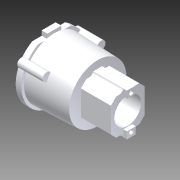
# Autodesk Inventor part: Gear housing BD drill motor
Saved by Autodesk Inventor 2012 (Build 160160000, 160)
## iProperties
Created: 2012-06-30
Part Number: Gear housing BD drill motor
Material: Default
Document SubType Name: Modeling
Designer: Bruce
Density: 1 g/cm^3
Author: Bruce
Autodesk Inventor part; units mm, degrees
ref_plane "YZ Plane" through (0, 0, 0) normal (1, 0, 0) x (0, 1, 0)
ref_plane "XZ Plane" through (0, 0, 0) normal (0, 1, 0) x (-1, 0, 0)
ref_plane "XY Plane" through (0, 0, 0) normal (0, 0, 1) x (1, 0, 0)
sketch "Sketch1" plane through (0, 0, 0) normal (0, 0, 1) x (1, 0, 0)
  line L0 (-46.094, 0) -> (-12.2454, 0)
  line L1 (-12.2454, 0) -> (-12.2454, 20.3708)
  line L2 (-12.2454, 20.3708) -> (-43.1064, 21.5265)
  line L3 (-43.1064, 21.5265) -> (-43.1064, 23.4315)
  line L4 (-43.1064, 23.4315) -> (-47.1704, 23.4315)
  line L5 (-47.1704, 23.4315) -> (-47.1704, 0)
  line L6 (-47.1704, 0) -> (-45.5559, 0)
  point P0 (0, 0)
  dimension "d0" = 4.064
  dimension "d1" = 1.905
  dimension "d2" = 23.4315
  dimension "d3" = 34.925
  dimension "d4" = 20.3708
  dimension "d15" = 0
  constraints: 14 end point, 2 parallel, 2 perpendicular, 1 horizontal, 1 point on line
  measures "d0" distance of L3.end L4.end
  measures "d1" distance of L2.end L3.end
  measures "d2" distance of L4.end L5.end
  measures "d3" distance between parallel lines of L1 L5
  measures "d4" distance of L0.end L1.end
  measures "d15" distance from line of point (0, 0) L0
revolve "Revolution1" add sketch "Sketch1" angle 360 about axis through (-46.094, 0, 0) along (1, 0, 0)
sketch "Sketch2" plane through (-47.1704, 0, 0) normal (-1, 0, 0) x (0, 0, 1)
  circle A0 centre (0, 0) radius 23.4315 projected
  circle A1 centre (0, 0) radius 22.3393 construction
  circle A2 centre (0, -22.3393) radius 3.048
  circle A3 centre (-19.355, 11.1548) radius 3.048
  circle A4 centre (19.355, 11.1548) radius 3.048
  circle A5 centre (-19.355, 11.1548) radius 1.6917
  circle A6 centre (19.355, 11.1548) radius 1.6917
  circle A7 centre (0, -22.3393) radius 1.7363
  line L0 (-11.6676, 20.32) -> (11.6676, 20.32)
  line L1 (11.6676, 20.32) -> (11.6676, 23.6728)
  line L2 (11.6676, 23.6728) -> (-11.6676, 23.6728)
  line L3 (-11.6676, 23.6728) -> (-11.6676, 20.32)
  line L4 (-4.9784, 20.32) -> (4.9784, 20.32)
  line L5 (4.9784, 20.32) -> (4.9784, 23.6728)
  line L6 (4.9784, 23.6728) -> (-4.9784, 23.6728)
  line L7 (-4.9784, 23.6728) -> (-4.9784, 20.32)
  line L8 (-4.9784, 23.6728) -> (4.9784, 23.6728)
  line L9 (4.9784, 23.6728) -> (4.9784, 20.32)
  line L10 (4.9784, 20.32) -> (-4.9784, 20.32)
  line L11 (-4.9784, 20.32) -> (-4.9784, 23.6728)
  dimension "d6" = 44.6786
  dimension "d7" = 6.096
  dimension "d8" = 6.096
  dimension "d9" = 6.096
  dimension "d10" = 38.6842
  dimension "d11" = 38.6842
  dimension "d12" = 38.71
  dimension "d16" = 20.32
  dimension "d17" = 9.9568
  dimension "d18" = 4.9784
  dimension "d19" = 3.3528
  constraints: 24 end point, 7 centre point, 6 parallel, 5 point on circle, 4 coincident, 4 collinear, 3 horizontal, 3 perpendicular, 2 point on line, 1 vertical alignment
  measures "d6" diameter of A1
  measures "d7" diameter of A4
  measures "d8" diameter of A3
  measures "d9" diameter of A2
  measures "d10" distance of A4.centre A2.centre
  measures "d11" distance of A3.centre A2.centre
  measures "d12" distance of A4.centre A3.centre
  measures "d16" distance from line of L0 A0.centre
  measures "d17" distance of L5.end L6.end
  measures "d18" distance from line of L7 A0.centre
  measures "d19" distance of L0.end L1.end
extrude "Extrusion1" add sketch "Sketch2" against normal blind 18.034 contours A4 A0 A6 | A0 A6 A4 | A2 A0 A7 | A0 A7 A2 | A6 A0 | A0 A6 | A7 A0 | A0 A7 | A3 A0 A5 | A0 A5 A3 | A5 A0 | A0 A5
extrude "Extrusion2" cut sketch "Sketch2" against normal blind 12.7 contours A6 A0 | A0 A6 | A7 A0 | A0 A7 | A5 A0 | A0 A5
extrude "Extrusion3" cut sketch "Sketch2" against normal blind 4.064 contours L0 L5 A0 | L5 L0 L7 A0 | L7 L0 A0
extrude "Extrusion4" add sketch "Sketch2" against normal blind 4.064 contours L5 L0 L7 A0 | A0 L7 L2 L5
sketch "Sketch3" plane through (-12.2454, 0, 0) normal (1, 0, 0) x (0, 0, -1)
  circle A0 centre (0, 0) radius 20.3708 projected
  line L0 (-12.0015, 12.7) -> (12.0015, 12.7)
  line L1 (12.0015, 12.7) -> (12.0015, -12.7)
  line L2 (12.0015, -12.7) -> (-12.0015, -12.7)
  line L3 (-12.0015, -12.7) -> (-12.0015, 12.7)
  line L4 (-3.175, 12.7) -> (3.175, 12.7)
  line L5 (3.175, 12.7) -> (3.175, 15.0495)
  line L6 (3.175, 15.0495) -> (-3.175, 15.0495)
  line L7 (-3.175, 15.0495) -> (-3.175, 12.7)
  line L8 (-3.175, -12.7) -> (3.175, -12.7)
  line L9 (3.175, -12.7) -> (3.175, -15.0495)
  line L10 (3.175, -15.0495) -> (-3.175, -15.0495)
  line L11 (-3.175, -15.0495) -> (-3.175, -12.7)
  dimension "d28" = 25.4
  dimension "d29" = 24.003
  dimension "d30" = 12.7
  dimension "d31" = 12.0015
  dimension "d32" = 2.3495
  dimension "d33" = 6.35
  dimension "d34" = 3.175
  dimension "d35" = 2.3495
  constraints: 24 end point, 6 parallel, 3 collinear, 3 horizontal, 3 perpendicular, 1 point on line
  measures "d28" distance of L0.end L1.end
  measures "d29" distance of L0.start L0.end
  measures "d30" distance from line of L0 A0.centre
  measures "d31" distance from line of L1 A0.centre
  measures "d32" distance of L4.end L5.end
  measures "d33" distance of L5.end L6.end
  measures "d34" distance from line of L7 A0.centre
  measures "d35" distance between parallel lines of L2 L10
extrude "Extrusion5" add sketch "Sketch3" along normal blind 23.876 contours L7 L6 L5 L0 | L2 L9 L10 L11
extrude "Extrusion6" add sketch "Sketch3" along normal blind 21.336 contours L0 L1 L2 L3
sketch "Sketch4" plane through (9.0906, 0, 0) normal (1, 0, 0) x (0, 0, -1)
  circle A0 centre (0, 0) radius 9.525
  dimension "d40" = 19.05
  constraints: 1 centre point, 1 coincident
  measures "d40" diameter of A0
extrude "Extrusion7" cut sketch "Sketch4" against normal blind 21.336
sketch "Sketch5" plane through (11.6306, 0, 0) normal (1, 0, 0) x (0, 0, -1)
  circle A0 centre (0, 0) radius 9.525 projected
  line L0 (-12.0015, 12.7) -> (-3.175, 12.7) projected
  line L1 (-12.0015, -12.7) -> (-12.0015, 12.7) projected
  line L2 (-3.175, -12.7) -> (-12.0015, -12.7) projected
  line L3 (3.175, -12.7) -> (-3.175, -12.7) projected
  line L4 (12.0015, -12.7) -> (3.175, -12.7) projected
  line L5 (12.0015, 12.7) -> (12.0015, -12.7) projected
  line L6 (3.175, 12.7) -> (12.0015, 12.7) projected
  line L7 (-3.175, 12.7) -> (3.175, 12.7) projected
  line L8 (-3.175, 12.7) -> (-3.175, 15.0495) projected
  line L9 (3.175, 15.0495) -> (3.175, 12.7) projected
  line L10 (-3.175, 15.0495) -> (3.175, 15.0495) projected
  line L11 (-3.175, 12.7) -> (3.175, 12.7)
  line L12 (3.175, 12.7) -> (3.175, 10.0457)
  line L13 (3.175, 10.0457) -> (-3.175, 10.0457)
  line L14 (-3.175, 10.0457) -> (-3.175, 12.7)
  line L15 (-3.175, -12.7) -> (3.175, -12.7)
  line L16 (3.175, -12.7) -> (3.175, -10.0457)
  line L17 (3.175, -10.0457) -> (-3.175, -10.0457)
  line L18 (-3.175, -10.0457) -> (-3.175, -12.7)
  line L19 (3.175, -15.0495) -> (-3.175, -15.0495) projected
  circle A1 centre (0, 11.9888) radius 1.4732
  circle A2 centre (0, -11.9888) radius 1.4732
  point P0 (0, 0)
  dimension "d43" = 11.9888
  dimension "d44" = 11.9888
  dimension "d52" = 5.0038
  dimension "d53" = 5.0038
  dimension "d56" = 2.9464
  dimension "d57" = 2.9464
  constraints: 16 end point, 4 parallel, 3 collinear, 2 centre point, 2 coincident, 2 horizontal, 2 perpendicular, 2 vertical alignment
  measures "d43" distance of point (0, 0) point (0, 11.989)
  measures "d44" distance of point (0, -11.989) point (0, 0)
  measures "d52" distance between parallel lines of L13 L10
  measures "d53" distance between parallel lines of L17 L19
  measures "d56" diameter of A1
  measures "d57" diameter of A2
extrude "Extrusion8" add sketch "Sketch5" against normal up to next contours L7 A1 L12 L13 L14 | L7 A1 | L18 L17 L16 L3 A2 | A2 L3 picked at (0.0552, 11.975) picked at (0.3662, -12.1358)
extrude "Extrusion9" cut sketch "Sketch5" against normal blind 21.336 contours A1 L7 | L7 A1 | A2 L3 | L3 A2
fillet "Fillet1" radius 3.175 4 edges at (-1.5774, 12.7, 3.175) (-1.5774, 12.7, -3.175) (-1.5774, -12.7, -3.175) (-1.5774, -12.7, 3.175)
chamfer "Chamfer1" distance 3.81 angle 45 4 edges at (-1.5774, 12.7, -12.0015) (-1.5774, 12.7, 12.0015) (-1.5774, -12.7, -12.0015) (-1.5774, -12.7, 12.0015)
equation "\"d8\" = d7"
equation "\"d9\" = d7"
equation "\"d11\" = d10"
equation "\"d18\" = 0.5 * d17"
equation "\"d30\" = 0.5 * d28"
equation "\"d31\" = 0.5 * d29"
equation "\"d34\" = 0.5 * d33"
equation "\"d35\" = d32"
equation "\"d44\" = d43"
equation "\"d57\" = d56"
body "Solid1"
